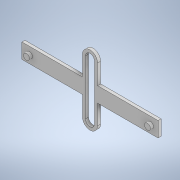
# Autodesk Inventor part: 축
Saved by Autodesk Inventor 2022 (Build 260153000, 153)
## iProperties
Created: 2022-10-28
Part Number: 축
Material: 일반
Document SubType Name: Modeling
Designer: whdls
Density: 1 g/cm^3
Appearance: 기본값
Author: whdls
Autodesk Inventor part; units mm, degrees
ref_plane "YZ Plane" through (0, 0, 0) normal (1, 0, 0) x (0, 1, 0)
ref_plane "XZ Plane" through (0, 0, 0) normal (0, 1, 0) x (-1, 0, 0)
ref_plane "XY Plane" through (0, 0, 0) normal (0, 0, 1) x (1, 0, 0)
sketch "스케치3" plane through (0, 0, 0) normal (0, 0, 1) x (1, 0, 0)
  line L0 (0, 9) -> (0, -9) construction
  line L1 (-1.5, 9) -> (-1.5, -9)
  line L2 (1.5, -9) -> (1.5, 9)
  arc A0 (1.5, 9) -> (-1.5, 9) centre (0, 9) ccw
  arc A1 (-1.5, -9) -> (1.5, -9) centre (0, -9) ccw
  line L3 (-2.5, 9) -> (-2.5, -9)
  arc A2 (-2.5, -9) -> (2.5, -9) centre (0, -9) ccw
  line L4 (2.5, -9) -> (2.5, 9)
  arc A3 (2.5, 9) -> (-2.5, 9) centre (0, 9) ccw
  line L5 (-3.5, 0) -> (3.5, 0) construction
  line L6 (0, -16.1) -> (0, 16.1) construction
  point P0 (0, 0)
  point P1 (0, 0)
  dimension "d8" = 18
  dimension "d9" = 1.5
  dimension "d10" = 1
  dimension "d11" = 9
  constraints: 12 end point, 8 point on circle, 4 centre point, 4 tangent, 2 parallel, 1 collinear, 1 midpoint, 1 vertical, 3 other
  measures "d8" distance of L0.start L0.end
  measures "d9" radius of A0
  measures "d10" distance between parallel lines of L2 L4
  measures "d11" distance from line of L5 L0.start
extrude "돌출3" add sketch "스케치3" along normal blind 1
sketch "스케치4" plane through (0, 0, 1) normal (0, 0, 1) x (1, 0, 0)
  line L0 (2.5, -9) -> (2.5, 9) projected
  line L1 (2.5, 2.5) -> (22.5, 2.5)
  line L2 (22.5, 2.5) -> (22.5, -2.5)
  line L3 (22.5, -2.5) -> (2.5, -2.5)
  line L4 (2.5, -2.5) -> (2.5, 2.5)
  point P0 (0, 0)
  point P1 (2.5, -2.5)
  dimension "d14" = 20
  dimension "d15" = 2.5
  dimension "d16" = 5
  constraints: 8 end point, 2 parallel, 1 horizontal, 1 perpendicular, 1 point on line
  measures "d14" distance of L1.start L1.end
  measures "d15" horizontal distance of point (0, 0) L1.start
  measures "d16" distance of L1.end L2.end
extrude "돌출4" add sketch "스케치4" against normal blind 1
sketch "스케치5" plane through (0, 0, 1) normal (0, 0, 1) x (1, 0, 0)
  circle A0 centre (20, 0) radius 1
  line L0 (-7.5, 0) -> (27.5, 0) construction
  line L1 (0, -16.1) -> (0, 16.1) construction
  point P0 (0, 0)
  dimension "d19" = 2
  dimension "d20" = 20
  constraints: 1 centre point, 1 point on line
  measures "d19" diameter of A0
  measures "d20" distance of point (0, 0) A0.centre
extrude "돌출5" add sketch "스케치5" along normal blind 1
mirror "미러1" about plane through (0, 0, 0) normal (1, 0, 0) of "돌출4", "돌출5"
